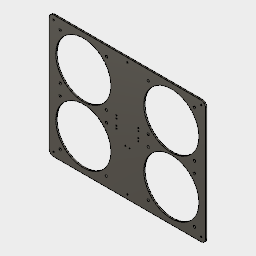
fan_mount (Autodesk Fusion 360 design; units mm, degrees)
Autodesk Fusion 360 part; units mm, degrees
sketch "sketch for fan hole pattern" plane through (0, 0, 0) normal (0, 0, 1) x (1, 0, 0)
  line L0 (0, 0) -> (355.6, 0)
  line L1 (355.6, 0) -> (355.6, 279.4)
  line L2 (355.6, 279.4) -> (0, 279.4)
  line L3 (0, 279.4) -> (0, 0)
  circle A0 centre (10, 269.4) radius 1.6
  circle A1 centre (345.6, 269.4) radius 1.6
  circle A2 centre (345.6, 10) radius 1.6
  circle A3 centre (10, 10) radius 1.6
  line L4 (25.3, 257.2) -> (130.3, 257.2) construction
  circle A4 centre (77.8, 204.7) radius 62.5
  circle A5 centre (130.3, 257.2) radius 2.5
  line L5 (25.3, 152.2) -> (130.3, 257.2) construction
  line L6 (130.3, 257.2) -> (130.3, 152.2) construction
  circle A6 centre (130.3, 152.2) radius 2.5
  line L7 (25.3, 152.2) -> (25.3, 257.2) construction
  line L8 (130.3, 152.2) -> (25.3, 257.2) construction
  line L9 (130.3, 152.2) -> (25.3, 152.2) construction
  circle A7 centre (25.3, 152.2) radius 2.5
  circle A8 centre (25.3, 257.2) radius 2.5
  circle A9 centre (225.3, 257.2) radius 2.5
  circle A10 centre (277.8, 204.7) radius 62.5
  circle A11 centre (330.3, 257.2) radius 2.5
  circle A12 centre (330.3, 152.2) radius 2.5
  circle A13 centre (225.3, 152.2) radius 2.5
  circle A14 centre (25.3, 127.2) radius 2.5
  circle A15 centre (77.8, 74.7) radius 62.5
  circle A16 centre (130.3, 127.2) radius 2.5
  circle A17 centre (130.3, 22.2) radius 2.5
  circle A18 centre (25.3, 22.2) radius 2.5
  circle A19 centre (225.3, 127.2) radius 2.5
  circle A20 centre (277.8, 74.7) radius 62.5
  circle A21 centre (330.3, 127.2) radius 2.5
  circle A22 centre (330.3, 22.2) radius 2.5
  circle A23 centre (225.3, 22.2) radius 2.5
  line L10 (77.8, 204.7) -> (277.8, 204.7) construction
  line L11 (277.8, 204.7) -> (277.8, 74.7) construction
  line L12 (277.8, 74.7) -> (77.8, 74.7) construction
  line L13 (77.8, 74.7) -> (77.8, 204.7) construction
  line L14 (177.8, 204.7) -> (177.8, 279.4) construction
  line L15 (277.8, 139.7) -> (355.6, 139.7) construction
  circle A24 centre (202.8, 152.7) radius 1.25
  circle A25 centre (202.8, 146.7) radius 1.25
  circle A26 centre (152.8, 146.7) radius 1.25
  circle A27 centre (152.8, 152.7) radius 1.25
  circle A28 centre (202.8, 126.7) radius 1.25
  circle A29 centre (202.8, 132.7) radius 1.25
  circle A30 centre (152.8, 126.7) radius 1.25
  circle A31 centre (152.8, 132.7) radius 1.25
  line L16 (177.8, 146.7) -> (177.8, 204.7) construction
  line L17 (152.8, 139.7) -> (77.8, 139.7) construction
  line L18 (202.8, 146.7) -> (152.8, 146.7) construction
  line L19 (152.8, 146.7) -> (152.8, 132.7) construction
  line L20 (152.8, 132.7) -> (202.8, 132.7) construction
  line L21 (202.8, 132.7) -> (202.8, 146.7) construction
  line L22 (277.8, 142.2) -> (212.16, 142.2) construction
  circle A32 centre (182.8, 102.7) radius 1.25
  circle A33 centre (172.8, 102.7) radius 1.25
  line L23 (182.8, 102.7) -> (172.8, 102.7) construction
  line L24 (177.8, 102.7) -> (177.8, 132.7) construction
  circle A34 centre (177.8, 269.4) radius 1.6
  circle A35 centre (177.8, 10) radius 1.6
  line L25 (10, 10) -> (345.6, 10) construction
  line L26 (345.6, 10) -> (345.6, 269.4) construction
  line L27 (345.6, 269.4) -> (10, 269.4) construction
  line L28 (10, 269.4) -> (10, 10) construction
  dimension "d1" = 355.6
  dimension "d2" = 279.4
  dimension "d4" = 10
  dimension "d5" = 3.2
  dimension "d11" = 105
  dimension "d12" = 5
  dimension "d13" = 125
  dimension "d16" = 200
  dimension "d17" = -130
  dimension "d23" = 335.6
  dimension "d24" = 259.4
  dimension "d25" = 2.5
  dimension "d26" = 6
  dimension "d29" = -50
  dimension "d30" = -20
  dimension "d31" = 2.5
  dimension "d32" = 10
  dimension "d33" = 30
  constraint horizontal L0
  constraint vertical L1
  constraint horizontal L2
  constraint vertical L3
  constraint coincident L0.start L3.end
  constraint equal A2 A3
  constraint equal A1 A2
  constraint equal A0 A1
  constraint perpendicular L7 L9
  constraint parallel L6 L7
  constraint horizontal L9
  constraint coincident L0.start L8
  constraint equal L6 L9
  constraint midpoint L0.start L5
  constraint equal A5 A8
  constraint equal A5 A6
  constraint equal A6 A7
  constraint horizontal L10
  constraint vertical L11
  constraint horizontal L12
  constraint vertical L13
  constraint midpoint L10 L0.start
  constraint midpoint L2
  constraint midpoint L11
  constraint midpoint L1
  constraint horizontal L15
  constraint vertical L14
  constraint equal A24 A25
  constraint vertical L0.start
  constraint midpoint L13
  constraint vertical L16
  constraint horizontal L17
  constraint horizontal L18
  constraint vertical L19
  constraint horizontal L20
  constraint vertical L21
  constraint coincident L19
  constraint coincident L18
  constraint midpoint L18
  constraint midpoint L19
  constraint coincident A10
  constraint tangent A10 L22
  constraint perpendicular L11 L22
  constraint equal A32 A33
  constraint horizontal L23
  constraint midpoint L23 L0.start
  constraint midpoint L20 L0.start
  constraint vertical L24
  constraint midpoint L27
  constraint midpoint L0.start L25
  constraint equal A34 A35
  constraint equal A0 A34
  measures "d2" distance of L0.start
  measures "d5" diameter of A0
  measures "d12" diameter of A8
  measures "d13" diameter of A4
  measures "d24" distance of L0.start
  measures "d25" diameter of A24
  measures "d26" distance of L0.start
  measures "d31" diameter of A32
extrude "Extrude1" add sketch "sketch for fan hole pattern" along normal blind 3
fillet "Fillet1" radius 10 4 edges at (355.6, 279.4, 1.5) (355.6, 0, 1.5) (0, 279.4, 1.5) (0, 0, 1.5)
ref_plane "WorkPlane1" through (177.8, 139.7, -20) normal (0, 0, -1) x (-1, 0, 0)
sketch "projected for cut" plane through (177.8, 139.7, -20) normal (0, 0, -1) x (1, 0, 0)
  circle A0 centre (-47.5, -12.5) radius 2.5
  circle A1 centre (-25, 7) radius 1.25
  circle A2 centre (47.5, 12.5) radius 2.5
  circle A3 centre (5, 37) radius 1.25
  circle A4 centre (0, -129.7) radius 1.6
  circle A5 centre (167.8, 129.7) radius 1.6
  circle A6 centre (-152.5, -12.5) radius 2.5
  circle A7 centre (-5, 37) radius 1.25
  circle A8 centre (-47.5, 12.5) radius 2.5
  circle A9 centre (100, 65) radius 62.5
  circle A10 centre (25, -7) radius 1.25
  circle A11 centre (0, 129.7) radius 1.6
  circle A12 centre (-47.5, -117.5) radius 2.5
  circle A13 centre (-25, -13) radius 1.25
  circle A14 centre (-25, -7) radius 1.25
  circle A15 centre (25, 7) radius 1.25
  circle A16 centre (25, 13) radius 1.25
  circle A17 centre (100, -65) radius 62.5
  circle A18 centre (-100, 65) radius 62.5
  circle A19 centre (-152.5, 12.5) radius 2.5
  circle A20 centre (152.5, 117.5) radius 2.5
  circle A21 centre (47.5, 117.5) radius 2.5
  circle A22 centre (-167.8, -129.7) radius 1.6
  circle A23 centre (152.5, -12.5) radius 2.5
  circle A24 centre (-152.5, -117.5) radius 2.5
  circle A25 centre (152.5, -117.5) radius 2.5
  circle A26 centre (47.5, -117.5) radius 2.5
  circle A27 centre (-25, 13) radius 1.25
  circle A28 centre (-167.8, 129.7) radius 1.6
  circle A29 centre (167.8, -129.7) radius 1.6
  circle A30 centre (152.5, 12.5) radius 2.5
  circle A31 centre (47.5, -12.5) radius 2.5
  circle A32 centre (-152.5, 117.5) radius 2.5
  circle A33 centre (-47.5, 117.5) radius 2.5
  circle A34 centre (25, -13) radius 1.25
  circle A35 centre (-100, -65) radius 62.5
  arc A36 (-167.8, 139.7) -> (-177.8, 129.7) centre (-167.8, 129.7) ccw
  line L0 (-177.8, 129.7) -> (-177.8, -129.7)
  arc A37 (-177.8, -129.7) -> (-167.8, -139.7) centre (-167.8, -129.7) ccw
  line L1 (-167.8, -139.7) -> (167.8, -139.7)
  arc A38 (167.8, -139.7) -> (177.8, -129.7) centre (167.8, -129.7) ccw
  line L2 (177.8, -129.7) -> (177.8, 129.7)
  arc A39 (177.8, 129.7) -> (167.8, 139.7) centre (167.8, 129.7) ccw
  line L3 (167.8, 139.7) -> (-167.8, 139.7)
